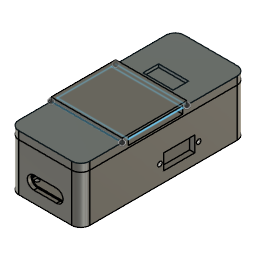
IMU (Autodesk Fusion 360 design; units mm, degrees)
Autodesk Fusion 360 part; units mm, degrees
sketch "草图1" plane through (0, 0, 0) normal (0, 0, 1) x (1, 0, 0)
  line L0 (-10, 20) -> (10, 20)
  line L1 (10, 20) -> (10, -20)
  line L2 (10, -20) -> (-10, -20)
  line L3 (-10, -20) -> (-10, 20)
  line L4 (0, 20) -> (0, -20) construction
  line L5 (-10, 10) -> (10, 10) construction
  circle A0 centre (-10, 10) radius 1.75
  circle A1 centre (10, 10) radius 1.75
  circle A2 centre (-10, 10) radius 1.25
  circle A3 centre (10, 10) radius 1.25
  line L6 (-10.1, -10) -> (10.1, -10) construction
  circle A4 centre (-10.1, -10) radius 2.5
  circle A5 centre (10.1, -10) radius 2.5
  circle A6 centre (0, -20) radius 1.25
  circle A7 centre (0, -20) radius 1.75
  circle A8 centre (0, 20) radius 1.75
  line L7 (-6, 18.2) -> (6, 18.2)
  line L8 (6, 18.2) -> (6, 13.2)
  line L9 (6, 13.2) -> (-6, 13.2)
  line L10 (-6, 13.2) -> (-6, 18.2)
  dimension "d1" = 20
  dimension "d2" = 40
  dimension "d4" = 20
  dimension "d5" = 10
  dimension "d6" = 20
  dimension "d7" = 10
  dimension "d8" = 3.5
  dimension "d9" = 3.5
  dimension "d10" = 2.5
  dimension "d11" = 2.5
  dimension "d12" = 20.2
  dimension "d13" = 10.1
  dimension "d14" = 5
  dimension "d15" = 5
  dimension "d16" = 10
  dimension "d17" = 2.5
  dimension "d18" = 3.5
  dimension "d19" = 3.5
  dimension "d20" = 12
  dimension "d21" = 5
  dimension "d22" = 6
  dimension "d23" = 1.8
  constraint horizontal L0
  constraint vertical L1
  constraint horizontal L2
  constraint vertical L3
  constraint midpoint L0 L4.start
  constraint midpoint L2 L4.end
  constraint horizontal L5
  constraint coincident L5.start A0.centre
  constraint coincident L5.end A1.centre
  constraint concentric A0 A2
  constraint concentric A1 A3
  constraint perpendicular L4 L6
  constraint coincident L6.start A4.centre
  constraint coincident L6.end A5.centre
  constraint coincident L4.end A6.centre
  constraint concentric A6 A7
  constraint coincident L4.start A8.centre
  constraint horizontal L7
  constraint vertical L8
  constraint horizontal L9
  constraint vertical L10
  measures "d1" distance of L0.start L0.end
  measures "d2" distance of L0.start L2.end
  measures "d4" vertical distance of origin L2.end
  measures "d5" distance of L0 L5
  measures "d6" distance of L5.start L5.end
  measures "d7" distance of L4 L5.start
  measures "d8" diameter of A0
  measures "d9" diameter of A1
  measures "d10" diameter of A2
  measures "d11" diameter of A3
  measures "d12" distance of L6.start L6.end
  measures "d13" distance of L4 L6.start
  measures "d14" diameter of A4
  measures "d15" diameter of A5
  measures "d16" distance of L2 L6
  measures "d17" diameter of A6
  measures "d18" diameter of A7
  measures "d19" diameter of A8
  measures "d20" distance of L7.start L7.end
  measures "d21" distance of L7.start L9.end
  measures "d22" distance of L4 L10
  measures "d23" distance of L0 L7
extrude "拉伸1" add sketch "草图1" along normal blind 3 contours L0 L1 L2 L3 A0 A1 A4 A5 A7 A8 | L1 A1 A3 | L1 A1 A3 | L3 A0 A2 | L3 A0 A2 | L2 A6 A7 | L2 A6 A7 makes body 1
extrude "拉伸2" add sketch "草图1" along normal blind 10 contours L7 L8 L9 L10 bodies 1
sketch "草图2" plane through (0, 0, 0) normal (0, 0, 1) x (1, 0, 0)
  line L0 (-12, 21) -> (12, 21)
  line L1 (12, 21) -> (12, -23)
  line L2 (12, -23) -> (-12, -23)
  line L3 (-12, -23) -> (-12, 21)
  circle A0 centre (-10, 10) radius 1.0823
  circle A1 centre (10, 10) radius 1.0591
  circle A2 centre (-10.1, -10) radius 2.4042
  circle A3 centre (10.1, -10) radius 2.4166
  circle A4 centre (0, -20) radius 1.1585
  line L4 (-10, 20) -> (10, 20)
  line L5 (10, 20) -> (10, -20)
  line L6 (10, -20) -> (-10, -20)
  line L7 (-10, -20) -> (-10, 20)
  line L8 (10.3, -20.3) -> (-10.3, -20.3)
  line L9 (-10.3, -20.3) -> (-10.3, 20.3)
  line L10 (-10.3, 20.3) -> (10.3, 20.3)
  line L11 (10.3, 20.3) -> (10.3, -20.3)
  line L12 (-13.1165, -25.5623) -> (-13.1165, 25.5623)
  line L13 (13.1165, 25.5623) -> (13.1165, -25.5623)
  line L14 (13.1165, -25.5623) -> (-13.1165, 25.5623) construction
  line L15 (-13.1165, -25.5623) -> (13.1165, 25.5623) construction
  line L16 (-13.1165, 22.0321) -> (13.1165, 22.0321)
  line L17 (-13.1165, -23.5106) -> (13.1165, -23.5106)
  dimension "d28" = -0.3
  constraint horizontal L0
  constraint vertical L1
  constraint horizontal L2
  constraint vertical L3
  constraint horizontal L4
  constraint vertical L5
  constraint horizontal L6
  constraint vertical L7
  constraint parallel L12 L13
  constraint coincident L14 origin
  constraint coincident L15 origin
  constraint coincident L12 L16.start
  constraint coincident L13 L16.end
  constraint perpendicular L13 L16
  constraint coincident L12 L17.start
  constraint coincident L13 L17.end
  constraint perpendicular L13 L17
extrude "拉伸3" add sketch "草图2" against normal blind 1.5 separate body contours L0 L1 L3 A0 A1 A2 A3 L9 L10 L11 | L3 A2 L9 | L1 A3 L11 | L1 L2 L3 A2 A3 A4 L8 L9 L11 | A0 A2 L7 L9 | A2 L7 L9 | A3 L5 L11 | A1 A3 L5 L11 | A2 A4 L6 L7 L8 L9 | A0 A1 A2 A3 A4 L4 L5 L6 L7 | A2 L7 | A0 L7 L9 | A0 L9 | A3 A4 L5 L6 L8 L11 | A3 L5 | A1 L11 | A1 L5 L11 | A0 L7 | A0 A1 L4 L5 L7 L9 L10 L11 | A1 L5 | A4 L8 | A4 L6 L8 | A4 L6 makes body 2
extrude "拉伸4" add sketch "草图2" along normal blind 1 contours L3 A2 L9 | L1 A3 L11 | A2 L7 L9 | A3 L5 L11 | A2 L7 | A0 L7 L9 | A0 L9 | A3 L5 | A1 L11 | A1 L5 L11 | A0 L7 | A1 L5 | A4 L8 | A4 L6 L8 | A4 L6 bodies 2
extrude "拉伸5" add sketch "草图2" along normal blind 6 and the other way blind 1.5 contours L3 A2 | L1 A3 | L12 L13 L16 L17 bodies 2
extrude "拉伸6" add 5 faces at (-10.521, -9.8562, 1) (0.8928, -19.8469, 1) (9.1946, -9.4156, 1) (10.2131, 9.9372, 1) (-10.1804, 10.3124, 1) along direction (0, 0, 1) blind 0.5 on bodies 2 bodies 2
sketch "草图3" plane through (0, 21, 0) normal (0, -1, 0) x (1, 0, 0)
  line L0 (-12, 0) -> (12, 0)
  line L1 (12, 0) -> (12, 6)
  line L2 (12, 6) -> (-12, 6)
  line L3 (-12, 6) -> (-12, 0)
  line L4 (0, 6) -> (0, 0) construction
  line L5 (-12, 6) -> (-11, 4.5)
  line L6 (-11, 4.5) -> (-12, 4.5)
  line L7 (11, 4.5) -> (12, 4.5)
  line L8 (12, 6) -> (11, 4.5)
  constraint midpoint L2 L4.start
  constraint coincident L4.end origin
  constraint coincident L2.end L3.start
  constraint coincident L3 L6.end
  constraint perpendicular L3 L6
  constraint symmetric L4 L2.end L1.end
  constraint symmetric L4 L5.end L7.start
  constraint symmetric L4 L6.end L7.end
extrude "拉伸7" add sketch "草图3" along normal blind 41 contours L3 L5 L6 | L1 L7 L8 bodies 2
extrude "拉伸8" cut sketch "草图3" along normal blind 12 contours L3 L5 L6 | L1 L7 L8 bodies 2
extrude "拉伸9" cut 2 faces at (-11.6667, -20, 5) (11.6667, -20, 5) along direction (0, 1, 0) blind 9 on bodies 2 bodies 2
sketch "草图4" plane through (0, 0, 6) normal (0, 0, 1) x (-1, 0, 0)
  line L0 (-12, 23) -> (12, 23)
  line L1 (12, 23) -> (12, 11)
  line L2 (12, 11) -> (12, -9)
  line L3 (12, -9) -> (12, -21)
  line L4 (12, -21) -> (-12, -21)
  line L5 (-12, -21) -> (-12, -9)
  line L6 (-12, -9) -> (-12, 11)
  line L7 (-12, 11) -> (-12, 23)
  line L8 (13.1165, -22.0321) -> (13.1165, 23.5106)
  line L9 (13.1165, 23.5106) -> (-13.1165, 23.5106)
  line L10 (-13.1165, 23.5106) -> (-13.1165, -22.0321)
  line L11 (-13.1165, -22.0321) -> (13.1165, -22.0321)
  line L12 (13.1165, -10.0589) -> (12, -10.0589)
  line L13 (12, -10.0589) -> (12, -9)
  line L14 (12, -9) -> (13.1165, -9)
  line L15 (13.1165, -9) -> (13.1165, -10.0589)
  line L16 (-12, -10) -> (-13.1165, -10)
  line L17 (-13.1165, -10) -> (-13.1165, -8.9928)
  line L18 (-13.1165, -8.9928) -> (-12, -8.9928)
  line L19 (-12, -8.9928) -> (-12, -10)
  line L20 (13.1165, 10.9187) -> (12, 10.9187)
  line L21 (12, 10.9187) -> (12, 12)
  line L22 (12, 12) -> (13.1165, 12)
  line L23 (13.1165, 12) -> (13.1165, 10.9187)
  line L24 (-12, 11) -> (-13.1165, 11)
  line L25 (-13.1165, 11) -> (-13.1165, 12.0535)
  line L26 (-13.1165, 12.0535) -> (-12, 12.0535)
  line L27 (-12, 12.0535) -> (-12, 11)
  constraint horizontal L12
  constraint vertical L13
  constraint horizontal L14
  constraint vertical L15
  constraint coincident L2.end L3.start
  constraint coincident L8 L12.start
  constraint horizontal L16
  constraint vertical L17
  constraint horizontal L18
  constraint vertical L19
  constraint coincident L10 L17.end
  constraint coincident L5 L16.start
  constraint horizontal L20
  constraint vertical L21
  constraint horizontal L22
  constraint vertical L23
  constraint coincident L1 L21.end
  constraint coincident L8 L20.start
  constraint horizontal L24
  constraint vertical L25
  constraint horizontal L26
  constraint vertical L27
  constraint coincident L10 L25.end
  constraint coincident L6.end L7.start
extrude "拉伸10" cut sketch "草图4" against normal blind 3 contours L7 L10 L24 L25 L26 L27 | L1 L2 L8 L20 L21 L22 L23 | L5 L6 L10 L16 L17 L18 L19 | L3 L8 L12 L13 L14 L15 bodies 2
sketch "草图5" plane through (0, 0, 0) normal (0, 0, 1) x (1, 0, 0)
  line L0 (12, 21) -> (-12, 21)
  line L1 (-12, 21) -> (-12, -23)
  line L2 (12, -23) -> (12, 21)
  line L3 (11.6151, 20.6151) -> (-11.6151, 20.6151)
  line L4 (-11.6151, 20.6151) -> (-11.6151, -22.6151)
  line L5 (-11.6151, -22.6151) -> (11.6151, -22.6151)
  line L6 (11.6151, -22.6151) -> (11.6151, 20.6151)
  line L7 (6, 18.2) -> (-6, 18.2)
  line L8 (-6, 18.2) -> (-6, 13.2)
  line L9 (-6, 13.2) -> (6, 13.2)
  line L10 (6, 13.2) -> (6, 18.2)
  line L11 (-6.4291, 18.6291) -> (-6.4291, 12.7709)
  line L12 (-6.4291, 12.7709) -> (6.4291, 12.7709)
  line L13 (6.4291, 12.7709) -> (6.4291, 18.6291)
  line L14 (6.4291, 18.6291) -> (-6.4291, 18.6291)
  point P0 (12, 21)
  point P1 (-12, -23)
  point P2 (6, 18.2)
  point P3 (-6, 13.2)
  dimension "d47" = -0.3849
  dimension "d48" = 0.4291
  constraint horizontal L0
  constraint vertical L1
  constraint vertical L2
  constraint coincident P1 L1.end
  constraint coincident P0 L0.start
  constraint horizontal L7
  constraint vertical L8
  constraint horizontal L9
  constraint vertical L10
  constraint coincident P3 L8.end
  constraint coincident P2 L7.start
extrude "拉伸11" add sketch "草图5" along normal blind 2 separate body contours L3 L4 L5 L6 makes body 3
move_body "移动1" bodies 3 to x (1, 0, 0) y (0, 1, 0) z (0, 0, 1) at (0, 0, 2)
move_body "移动2" bodies 3 to x (1, 0, 0) y (0, 1, 0) z (0, 0, 1) at (0, 0, 13)
extrude "拉伸12" cut 1 faces at (2.143, -10.8198, 17) along direction (0, 0, -1) blind 0.7 on bodies 3 bodies 3
move_body "移动3" bodies 3 to x (1, 0, 0) y (0, 1, 0) z (0, 0, 1) at (0, 0, -12)
extrude "拉伸13" add 1 faces at (11.6151, -8.205, 3.4333) along direction (1, 0, 0) blind 0.3 on bodies 3 bodies 3
extrude "拉伸14" cut 4 faces at (-12.3722, 9.353, 3) (-12.3722, -11.6396, 3) (12.3722, -11.7023, 3) (12.7443, 9.3286, 3) along direction (0, 0, -1) blind 3 on bodies 2 bodies 2
sketch "草图6" plane through (0, 0, 4.3) normal (0, 0, 1) x (-1, 0, 0)
  line L0 (6.4291, -18.6291) -> (-6.4291, -18.6291)
  line L1 (-6.4291, -18.6291) -> (-6.4291, -12.7709)
  line L2 (-6.4291, -12.7709) -> (6.4291, -12.7709)
  line L3 (6.4291, -12.7709) -> (6.4291, -18.6291)
  line L4 (-11.9151, -20.6151) -> (11.6151, -20.6151)
  line L5 (11.6151, -20.6151) -> (11.6151, 22.6151)
  line L6 (11.6151, 22.6151) -> (-11.9151, 22.6151)
  line L7 (-11.9151, 22.6151) -> (-11.9151, -20.6151)
  line L8 (9, -8) -> (-8.9143, -8)
  line L9 (-8.9143, -8) -> (-8.9143, 14.5)
  line L10 (-8.9143, 14.5) -> (9, 14.5)
  line L11 (9, 14.5) -> (9, -8)
  dimension "d57" = 22.5
  constraint horizontal L8
  constraint vertical L9
  constraint horizontal L10
  constraint vertical L11
  measures "d57" distance of L8.start L10.end
extrude "拉伸15" add sketch "草图6" along normal blind 6.5 contours L8 L9 L10 L11 bodies 3
fillet "圆角1" radius 1 8 edges at (-0.0428, 8, 10.8) (-0.0428, -14.5, 10.8) (-9, -3.25, 10.8) (8.9143, -3.25, 10.8) (-9, 8, 7.55) (-9, -14.5, 7.55) (8.9143, -14.5, 7.55) (8.9143, 8, 7.55) on bodies 3
sketch "草图7" plane through (-9, 0, 0) normal (-1, 0, 0) x (0, -1, 0)
  line L0 (13.5, 4.3) -> (13.5, 9.8)
  line L1 (13.5, 9.8) -> (-7, 9.8)
  line L2 (-7, 9.8) -> (-7, 4.3)
  line L3 (-7, 4.3) -> (13.5, 4.3)
  line L4 (-7, 9.8) -> (13.5, 9.8)
  line L5 (13.5, 9.8) -> (13.5, 6.8)
  line L6 (13.5, 6.8) -> (-7, 6.8)
  line L7 (-7, 6.8) -> (-7, 9.8)
  dimension "d62" = 3
  constraint horizontal L4
  constraint vertical L5
  constraint horizontal L6
  constraint vertical L7
  constraint coincident L0 L5.end
  constraint coincident L1.end L2.start
  measures "d62" distance of L1.end L6.end
extrude "拉伸16" cut sketch "草图7" against normal blind 20 contours L0 L1 L2 L4 L5 L6 L7 bodies 3
fillet "圆角2" radius 0.5 4 edges at (-9, -3.25, 9.8) (-9, -3.25, 6.8) (8.9143, -3.25, 9.8) (8.9143, -3.25, 6.8) on bodies 3
sketch "草图8" plane through (0, 0, 0) normal (0, 0, 1) x (1, 0, 0)
  line L0 (75, 20) -> (98.5, 20)
  line L1 (98.5, 20) -> (98.5, -41)
  line L2 (98.5, -41) -> (75, -41)
  line L3 (75, -41) -> (75, 20)
  line L4 (75, 19) -> (98.5, 19)
  line L5 (74, 20) -> (74, -42)
  line L6 (74, -42) -> (99.5, -42)
  line L7 (99.5, -42) -> (99.5, 20)
  line L8 (99.5, 20) -> (74, 20)
  dimension "d67" = 23.5
  dimension "d68" = 61
  constraint horizontal L0
  constraint vertical L1
  constraint horizontal L2
  constraint vertical L3
  constraint coincident L3 L4.start
  constraint coincident L1 L4.end
  constraint perpendicular L1 L4
  constraint perpendicular L0 L5
  constraint perpendicular L5 L6
  constraint perpendicular L6 L7
  constraint perpendicular L5 L8
  measures "d67" distance of L0.start L0.end
  measures "d68" distance of L0.start L2.end
extrude "拉伸17" add sketch "草图8" along normal blind 21 separate body contours L0 L1 L3 L4 L8 | L1 L2 L3 L5 L6 L7 L8 makes body 4
extrude "拉伸18" add sketch "草图8" along normal blind 2 contours L1 L2 L3 L4 bodies 4
sketch "草图9" plane through (0, 0, 0) normal (0, 1, 0) x (1, 0, 0)
  line L0 (105, -1) -> (122.5, -1)
  line L1 (122.5, -1) -> (122.5, 0)
  line L2 (122.5, 0) -> (105, 0)
  line L3 (105, 0) -> (105, -1)
  line L4 (109.35, -3.9902) -> (118.15, -3.9902)
  arc A0 (118.15, -3.9902) -> (118.15, -0.9902) centre (118.15, -2.4902) ccw
  line L5 (118.15, -0.9902) -> (109.35, -0.9902)
  arc A1 (109.35, -0.9902) -> (109.35, -3.9902) centre (109.35, -2.4902) ccw
  line L6 (109.35, -2.4902) -> (118.15, -2.4902) construction
  point P0 (113.75, -1)
  point P1 (113.75, -2.4902)
  dimension "d73" = 17.5
  dimension "d76" = 3
  constraint horizontal L0
  constraint vertical L1
  constraint horizontal L2
  constraint vertical L3
  constraint midpoint L0 P0
  constraint tangent L4 A0
  constraint tangent A0 L5
  constraint parallel L4 L5
  constraint tangent L5 A1
  constraint tangent L4 A1
  constraint parallel L0 L6
  constraint midpoint L6 P1
  measures "d73" distance of L0.start L0.end
  measures "d76" diameter of A0
extrude "拉伸19" add sketch "草图9" along normal blind 28 separate body contours L0 L1 L2 L3 A0 L5 A1 | L0 A0 L5 A1 makes body 5
extrude "拉伸20" add sketch "草图9" along normal blind 6.1 and the other way blind 0.7 contours L0 L4 A0 A1 bodies 5
sketch "草图10" plane through (0, 0, 1) normal (0, 0, 1) x (-1, 0, 0)
  line L0 (-118.3209, -6.1) -> (-118.3209, 0)
  line L1 (-118.3209, 0) -> (-122.5, 0)
  line L2 (-122.5, 0) -> (-122.5, -28)
  line L3 (-122.5, -28) -> (-105, -28)
  line L4 (-105, -28) -> (-105, 0)
  line L5 (-105, 0) -> (-109.1791, 0)
  line L6 (-109.1791, 0) -> (-109.1791, -6.1)
  line L7 (-109.1791, -6.1) -> (-118.3209, -6.1)
  line L8 (-120.75, -1.9) -> (-106.75, -1.9)
  circle A0 centre (-106.75, -1.9) radius 0.8
  circle A1 centre (-120.75, -1.9) radius 0.8
  line L9 (-105, 0) -> (-122.5, 0)
  dimension "d81" = 14
  dimension "d82" = 1.75
  dimension "d83" = 1.6
  dimension "d84" = 1.6
  dimension "d87" = 17.5
  dimension "d91" = 1.9
  constraint perpendicular L4 L8
  constraint coincident L8.end A0.centre
  constraint coincident L8.start A1.centre
  measures "d81" distance of L8.start L8.end
  measures "d82" distance of L2 L8.start
  measures "d83" diameter of A0
  measures "d84" diameter of A1
  measures "d87" distance of L2.end L3.end
  measures "d91" distance of L8 L9
extrude "拉伸21" cut sketch "草图10" against normal blind 1.6 contours A0 | A1 bodies 5
sketch "草图11" plane through (0, 0, 2) normal (0, 0, 1) x (-1, 0, 0)
  line L0 (-75, -19) -> (-75, 41)
  line L1 (-75, 41) -> (-98.5, 41)
  line L2 (-98.5, 41) -> (-98.5, -19)
  line L3 (-98.5, -19) -> (-75, -19)
  line L4 (-86.75, 41) -> (-86.75, -19) construction
  line L5 (-95.5, 41) -> (-78, 41)
  line L6 (-78, 41) -> (-78, 22.3)
  line L7 (-78, 22.3) -> (-95.5, 22.3)
  line L8 (-95.5, 22.3) -> (-95.5, 41)
  line L9 (-93.75, 39.1) -> (-79.75, 39.1) construction
  circle A0 centre (-93.75, 39.1) radius 0.5239
  circle A1 centre (-79.75, 39.1) radius 0.5069
  dimension "d88" = 17.5
  dimension "d89" = 18.7
  dimension "d90" = 8.75
  dimension "d92" = 14
  dimension "d93" = 1.75
  dimension "d94" = 1.9
  constraint midpoint L1 L4.start
  constraint midpoint L3 L4.end
  constraint horizontal L5
  constraint vertical L6
  constraint horizontal L7
  constraint vertical L8
  constraint coincident L1 L5.start
  constraint parallel L1 L9
  constraint coincident L9.start A0.centre
  constraint coincident L9.end A1.centre
  measures "d88" distance of L5.start L5.end
  measures "d89" distance of L5.start L7.end
  measures "d90" distance of L4 L8
  measures "d92" distance of L9.start L9.end
  measures "d93" distance of L8 L9.start
  measures "d94" distance of L5 L9
extrude "拉伸22" add sketch "草图11" along normal blind 2.5 contours L1 L5 L6 L7 L8 bodies 4
thread "螺纹1" "ISO Metric profile 2.0 M2x0.4 M2x0.4 6H" major diameter 2.074 minor diameter 1.623 pitch 0.4 angle 60 resizes the face on face at (93.4658, -39.5401, 3.6667) on face at (79.4146, -39.48, 3.6667) on bodies 4
move_body "移动4" bodies 5 to x (1, 0, 0) y (0, 1, 0) z (0, 0, 1) at (-26.9998, -40.9666, 1.427)
move_body "移动5" bodies 5 to x (1, 0, 0) y (0, 1, 0) z (0, 0, 1) at (0, 0, 3.1)
sketch "草图12" plane through (0, -41, 0) normal (0, 1, 0) x (-1, 0, 0)
  line L0 (-78, 4.5) -> (-78, 2)
  line L1 (-78, 2) -> (-75, 2)
  line L2 (-75, 2) -> (-75, 21)
  line L3 (-75, 21) -> (-98.5, 21)
  line L4 (-98.5, 21) -> (-98.5, 2)
  line L5 (-98.5, 2) -> (-95.5, 2)
  line L6 (-95.5, 2) -> (-95.5, 4.5)
  line L7 (-95.5, 4.5) -> (-78, 4.5)
  arc A0 through (-91.1502, 8.5172, -0.6666) (-92.6478, 7.1028, -0.6666) (-91.3212, 5.527, -0.6666)
  arc A1 through (-82.1793, 5.527, -0.6666) (-80.8527, 7.1028, -0.6666) (-82.3503, 8.5172, -0.6666)
  line L8 (-91.1502, 8.5172, -0.6666) -> (-82.3503, 8.5172, -0.6666)
  line L9 (-91.3212, 5.527, -0.6666) -> (-82.1793, 5.527, -0.6666)
  line L10 (-91.1503, 5.3759) -> (-82.35, 5.3759)
  arc A2 (-82.35, 5.3759) -> (-82.35, 8.6585) centre (-82.35, 7.0172) ccw
  line L11 (-82.35, 8.6585) -> (-91.1503, 8.6585)
  arc A3 (-91.1503, 8.6585) -> (-91.1503, 5.3759) centre (-91.1503, 7.0172) ccw
  line L12 (-91.1503, 7.0172) -> (-82.35, 7.0172) construction
  line L13 (-82.35, 9.5343) -> (-91.1503, 9.5343)
  arc A4 (-91.1503, 9.5343) -> (-91.1503, 4.5) centre (-91.1503, 7.0172) ccw
  line L14 (-91.1503, 4.5) -> (-82.35, 4.5)
  arc A5 (-82.35, 4.5) -> (-82.35, 9.5343) centre (-82.35, 7.0172) ccw
  line L15 (-82.35, 7.0172) -> (-91.1503, 7.0172) construction
  constraint tangent L10 A2
  constraint tangent A2 L11
  constraint parallel L10 L11
  constraint tangent L11 A3
  constraint tangent L10 A3
  constraint horizontal L12
  constraint tangent L13 A4
  constraint tangent A4 L14
  constraint parallel L13 L14
  constraint tangent L14 A5
  constraint tangent L13 A5
  constraint coincident A3.centre L12.start
  constraint parallel L12 L15
  constraint coincident A2.centre L12.end
extrude "拉伸23" cut sketch "草图12" against normal blind 3 contours L10 A2 L11 A3 bodies 4
sketch "草图13" plane through (0, -42, 0) normal (0, -1, 0) x (1, 0, 0)
  line L0 (91.1503, 5.3759) -> (82.35, 5.3759)
  arc A0 (82.35, 8.6585) -> (82.35, 5.3759) centre (82.35, 7.0172) ccw
  line L1 (82.35, 8.6585) -> (91.1503, 8.6585)
  arc A1 (91.1503, 5.3759) -> (91.1503, 8.6585) centre (91.1503, 7.0172) ccw
  line L2 (74, 0) -> (99.5, 0)
  line L3 (99.5, 0) -> (99.5, 21)
  line L4 (99.5, 21) -> (74, 21)
  line L5 (74, 21) -> (74, 0)
  line L6 (82.35, 4.5) -> (91.1503, 4.5)
  arc A2 (91.1503, 4.5) -> (91.1503, 9.5343) centre (91.1503, 7.0172) ccw
  line L7 (91.1503, 9.5343) -> (82.35, 9.5343)
  arc A3 (82.35, 9.5343) -> (82.35, 4.5) centre (82.35, 7.0172) ccw
  line L8 (82.35, 7.0172) -> (91.1503, 7.0172) construction
  constraint tangent L6 A2
  constraint tangent A2 L7
  constraint parallel L6 L7
  constraint tangent L7 A3
  constraint tangent L6 A3
  constraint coincident A1.centre A2.centre
  constraint horizontal L8
  constraint coincident A0.centre A3.centre
extrude "拉伸24" cut sketch "草图13" against normal blind 0.5 contours L6 A2 L7 A3 bodies 4
sketch "草图14" plane through (0, 0, 0) normal (0, 0, 1) x (1, 0, 0)
  line L0 (50, 5) -> (70, 5)
  line L1 (70, 5) -> (70, -47.6)
  line L2 (70, -47.6) -> (50, -47.6)
  line L3 (50, -47.6) -> (50, 5)
  circle A0 centre (52, 3) radius 1.05
  circle A1 centre (68, 3) radius 1.05
  line L4 (55, 5) -> (65, 5)
  line L5 (65, 5) -> (65, 12.7)
  line L6 (65, 12.7) -> (55, 12.7)
  line L7 (55, 12.7) -> (55, 5)
  dimension "d103" = 20
  dimension "d104" = 52.6
  dimension "d105" = 2.1
  dimension "d106" = 2.1
  dimension "d107" = 2
  dimension "d108" = 2
  dimension "d109" = 2
  dimension "d110" = 2
  dimension "d111" = 10
  dimension "d112" = 7.7
  dimension "d113" = 5
  constraint horizontal L0
  constraint vertical L1
  constraint horizontal L2
  constraint vertical L3
  constraint horizontal L4
  constraint vertical L5
  constraint horizontal L6
  constraint vertical L7
  constraint coincident L0 L4.start
  measures "d103" distance of L0.start L0.end
  measures "d104" distance of L0.start L2.end
  measures "d105" diameter of A0
  measures "d106" diameter of A1
  measures "d107" distance of L0 A1.centre
  measures "d108" distance of L0 A0.centre
  measures "d109" distance of L3 A0.centre
  measures "d110" distance of L1 A1.centre
  measures "d111" distance of L4.start L4.end
  measures "d112" distance of L4.start L6.end
  measures "d113" distance of L3 L7
extrude "拉伸25" add sketch "草图14" along normal blind 1.4 separate body contours L0 L1 L2 L3 L4 makes body 6
extrude "拉伸26" add sketch "草图14" along normal blind 4.2 and the other way blind 0.6 contours L0 L4 L5 L6 L7 bodies 6
sketch "草图15" plane through (0, 0, 1.4) normal (0, 0, 1) x (-1, 0, 0)
  circle A0 centre (-68, -3) radius 1.05
  circle A1 centre (-52, -3) radius 1.05
  line L0 (-70, -5) -> (-65, -5)
  line L1 (-65, -5) -> (-55, -5)
  line L2 (-55, -5) -> (-50, -5)
  line L3 (-50, -5) -> (-50, 47.6)
  line L4 (-50, 47.6) -> (-70, 47.6)
  line L5 (-70, 47.6) -> (-70, -5)
  line L6 (-54.7, 2.1) -> (-65.3, 2.1)
  line L7 (-65.3, 2.1) -> (-65.3, 7.1)
  line L8 (-65.3, 7.1) -> (-54.7, 7.1)
  line L9 (-54.7, 7.1) -> (-54.7, 2.1)
  line L10 (-50, -5) -> (-70, -5)
  line L11 (-70, -5) -> (-70, 47.6)
  line L12 (-50, 47.6) -> (-50, -5)
  dimension "d120" = 10.6
  dimension "d121" = 5
  dimension "d122" = 7.1
  dimension "d123" = 4.7
  dimension "d124" = 4.7
  constraint horizontal L6
  constraint vertical L7
  constraint horizontal L8
  constraint vertical L9
  measures "d120" distance of L6.start L6.end
  measures "d121" distance of L6.start L8.end
  measures "d122" distance of L6 L10
  measures "d123" distance of L7 L11
  measures "d124" distance of L9 L12
extrude "拉伸27" add sketch "草图15" along normal blind 8.4 contours L6 L7 L8 L9 bodies 6
move_body "移动6" bodies 6 to x (1, 0, 0) y (0, 1, 0) z (0, 0, 1) at (27, 8, 11)
sketch "草图16" plane through (0, -41, 0) normal (0, 1, 0) x (-1, 0, 0)
  line L0 (-98.5, 21) -> (-98.5, 2) construction
  line L1 (-75, 2) -> (-75, 21) construction
  line L2 (-98.5, 11) -> (-75, 11) construction
  line L3 (-98.5, 2) -> (-95.5, 2) construction
  line L4 (-98.5, 11) -> (-96.1003, 11)
  line L5 (-96.1003, 11) -> (-96.1003, 9)
  line L6 (-96.1003, 9) -> (-98.5, 9)
  line L7 (-98.5, 9) -> (-98.5, 11)
  line L8 (-98.5, 12.5) -> (-96.1003, 12.5)
  line L9 (-96.1003, 12.5) -> (-96.1003, 14.5)
  line L10 (-96.1003, 14.5) -> (-98.5, 14.5)
  line L11 (-98.5, 14.5) -> (-98.5, 12.5)
  line L12 (-75, 11) -> (-77.5, 11)
  line L13 (-77.5, 11) -> (-77.5, 9)
  line L14 (-77.5, 9) -> (-75, 9)
  line L15 (-75, 9) -> (-75, 11)
  line L16 (-75, 12.5) -> (-77.5, 12.5)
  line L17 (-77.5, 12.5) -> (-77.5, 14.5)
  line L18 (-77.5, 14.5) -> (-75, 14.5)
  line L19 (-75, 14.5) -> (-75, 12.5)
  dimension "d127" = 9
  dimension "d128" = 2
  dimension "d129" = 2
  dimension "d130" = 1.5
  dimension "d138" = 1.5
  constraint coincident L0 L2.start
  constraint coincident L1 L2.end
  constraint perpendicular L1 L2
  constraint horizontal L4
  constraint vertical L5
  constraint horizontal L6
  constraint vertical L7
  constraint horizontal L8
  constraint vertical L9
  constraint horizontal L10
  constraint vertical L11
  constraint coincident L0 L8.start
  constraint horizontal L12
  constraint vertical L13
  constraint horizontal L14
  constraint vertical L15
  constraint horizontal L16
  constraint vertical L17
  constraint horizontal L18
  constraint vertical L19
  constraint coincident L1 L16.start
  measures "d127" distance of L2 L3
  measures "d128" distance of L2.start L6.end
  measures "d129" distance of L8.start L10.end
  measures "d130" distance of L2 L8
  measures "d138" distance of L12 L16
extrude "拉伸28" add sketch "草图16" along normal blind 3 bodies 4
move_face "偏移面1" offset -1 4 faces at (85.2834, -41.1667, 8.6585) (91.7878, -41.1667, 5.5047) (81.7886, -41.3333, 5.4748) (88.2168, -41.1667, 5.3759) on bodies 4
extrude "拉伸29" add 4 faces at (97.7001, -38, 13.8333) (96.9002, -38, 9.6667) (75.8333, -38, 13.1667) (76.6667, -38, 10.3333) along direction (0, 1, 0) blind 1 on bodies 4 bodies 4
extrude "拉伸30" cut 2 faces at (97.7001, -37, 13.8333) (75.8333, -37, 13.1667) along direction (0, -1, 0) blind 4 on bodies 4 bodies 4
extrude "拉伸31" add sketch "草图16" along normal blind 4 contours L8 L9 L10 L11 | L16 L17 L18 L19 bodies 4
sketch "草图17" plane through (0, 0, 2) normal (0, 0, 1) x (-1, 0, 0)
  line L0 (-78, 41) -> (-78, 22.3)
  line L1 (-78, 22.3) -> (-95.5, 22.3)
  line L2 (-95.5, 22.3) -> (-95.5, 41)
  line L3 (-95.5, 41) -> (-98.5, 41)
  line L4 (-98.5, 41) -> (-98.5, -19)
  line L5 (-98.5, -19) -> (-75, -19)
  line L6 (-75, -19) -> (-75, 41)
  line L7 (-75, 41) -> (-78, 41)
  circle A0 centre (-95, -11) radius 1.05
  circle A1 centre (-79, -11) radius 1.05
  line L8 (-98.5, -8.2706, -2) -> (-94.3, -8.2706, -2)
  line L9 (-93.2, -9.3706, -2) -> (-93.2, -11.4, -2)
  line L10 (-94.3, -12.5, -2) -> (-98.5, -12.5, -2)
  line L11 (-98.5, -12.5, -2) -> (-98.5, -8.2706, -2)
  line L12 (-98.5, -20, -2) -> (-98.5, 41, -2)
  line L13 (-75, -8.2706, -2) -> (-80.3, -8.2706, -2)
  line L14 (-81.4, -9.3706, -2) -> (-81.4, -11.4, -2)
  line L15 (-80.3, -12.5, -2) -> (-75, -12.5, -2)
  line L16 (-75, -12.5, -2) -> (-75, -8.2706, -2)
  line L17 (-75, 41, -2) -> (-75, -20, -2)
  arc A2 through (-93.2, -9.3706, -2) (-93.5222, -8.5928, -2) (-94.3, -8.2706, -2)
  arc A3 through (-94.3, -12.5, -2) (-93.5222, -12.1778, -2) (-93.2, -11.4, -2)
  arc A4 through (-80.3, -8.2706, -2) (-81.0778, -8.5928, -2) (-81.4, -9.3706, -2)
  arc A5 through (-81.4, -11.4, -2) (-81.0778, -12.1778, -2) (-80.3, -12.5, -2)
  dimension "d141" = 1.1
extrude "拉伸32" add sketch "草图17" along normal blind 11 contours L8 L9 L10 L11 L12 A2 A3 | L13 L14 L15 L16 L17 A4 A5 in plane through (0, 0, 0) normal (0, 0, 1) bodies 4
extrude "拉伸33" cut sketch "草图17" along normal blind 9 contours A0 | A1 bodies 4
thread "螺纹2" "ISO Metric profile 2.0 M2x0.25 M2x0.25 6H" major diameter 2.0555 minor diameter 1.7694 pitch 0.25 angle 60 resizes the face on face at (95.837, 11.634, 8) on face at (79.837, 11.634, 8) on bodies 4
sketch "草图18" plane through (0, 19, 0) normal (0, -1, 0) x (1, 0, 0)
  line L0 (75, 2) -> (98.5, 2)
  line L1 (98.5, 2) -> (98.5, 21)
  line L2 (98.5, 21) -> (75, 21)
  line L3 (75, 21) -> (75, 2)
  line L4 (82, 12.4) -> (92, 12.4)
  line L5 (92, 12.4) -> (92, 15.2)
  line L6 (92, 15.2) -> (82, 15.2)
  line L7 (82, 15.2) -> (82, 12.4)
  line L8 (81.8034, 12.2034) -> (92.1966, 12.2034)
  line L9 (92.1966, 12.2034) -> (92.1966, 15.3966)
  line L10 (92.1966, 15.3966) -> (81.8034, 15.3966)
  line L11 (81.8034, 15.3966) -> (81.8034, 12.2034)
  dimension "d148" = 0.1966
extrude "拉伸34" cut sketch "草图18" against normal blind 2.5 contours L4 L5 L6 L7 | L8 L9 L10 L11 bodies 4
move_face "偏移面2" offset -0.4 4 faces at (88.7322, 19.3333, 15.3966) (81.8034, 19.3333, 14.3322) (85.2678, 19.3333, 12.2034) (92.1966, 19.3333, 13.2678) on bodies 4
sketch "草图19" plane through (0, 0, 21) normal (0, 0, 1) x (-1, 0, 0)
  line L0 (-75, 41) -> (-75, -19)
  line L1 (-75, -19) -> (-98.5, -19)
  line L2 (-98.5, -19) -> (-98.5, 41)
  line L3 (-98.5, 41) -> (-75, 41)
  line L4 (-99.5, -20) -> (-74, -20)
  line L5 (-74, -20) -> (-74, 42)
  line L6 (-74, 42) -> (-99.5, 42)
  line L7 (-99.5, 42) -> (-99.5, -20)
  circle A0 centre (-95.5585, 38) radius 2.05
  circle A1 centre (-77.7898, -16.3705) radius 2.05
  line L8 (-75, -19) -> (-81, -19)
  line L9 (-81, -19) -> (-81, -13)
  line L10 (-81, -13) -> (-75, -13)
  line L11 (-75, -13) -> (-75, -19)
  line L12 (-98.5, 41) -> (-92.5, 41)
  line L13 (-92.5, 41) -> (-92.5, 35)
  line L14 (-92.5, 35) -> (-98.5, 35)
  line L15 (-98.5, 35) -> (-98.5, 41)
  point P0 (-96, 38)
  dimension "d152" = 4.1
  dimension "d153" = 4.1
  dimension "d154" = 6
  dimension "d155" = 6
  dimension "d156" = 6
  dimension "d157" = 6
  constraint horizontal L8
  constraint vertical L9
  constraint horizontal L10
  constraint vertical L11
  constraint coincident L0.end L1.start
  constraint horizontal L12
  constraint vertical L13
  constraint horizontal L14
  constraint vertical L15
  constraint coincident L2.end L3.start
  measures "d152" diameter of A0
  measures "d153" diameter of A1
  measures "d154" distance of L0.end L8.end
  measures "d155" distance of L0.end L10.end
  measures "d156" distance of L2.end L12.end
  measures "d157" distance of L2.end L14.end
extrude "拉伸35" add sketch "草图19" against normal blind 3 contours L2 L3 L12 L13 L14 L15 | A0 bodies 4
extrude "拉伸36" add sketch "草图19" against normal blind 3 contours L0 L1 L8 L9 L10 L11 | A1 bodies 4
extrude "拉伸37" cut sketch "草图19" against normal blind 2.1 contours A0 | A1 bodies 4
fillet "圆角3" radius 2.5 2 edges at (92.5, -35, 19.5) (81, 13, 19.5) on bodies 4
extrude "拉伸38" add 1 faces at (99.5, -21.3333, 14) along direction (1, 0, 0) blind 1 on bodies 4 bodies 4
extrude "拉伸39" add 1 faces at (89.0322, 20, 3.9345) along direction (0, 1, 0) blind 1 on bodies 4 bodies 4
extrude "拉伸40" add 1 faces at (74, -21, 14) along direction (-1, 0, 0) blind 1 on bodies 4 bodies 4
extrude "拉伸41" add 1 faces at (85.2833, -42, 17.1781) along direction (0, -1, 0) blind 1 on bodies 4 bodies 4
extrude "拉伸42" cut 1 faces at (99.8333, -19, 21) along direction (0, 0, -1) blind 2.5 on bodies 4 bodies 4
extrude "拉伸43" cut sketch "草图19" against normal blind 3 contours L2 L3 L12 L13 L14 L15 | A0 bodies 4
extrude "拉伸44" cut sketch "草图19" against normal blind 3 contours L0 L1 L8 L9 L10 L11 | A1 bodies 4
extrude "拉伸45" add sketch "草图19" against normal blind 5.5 contours L0 L1 L8 L9 L10 L11 | L2 L3 L12 L13 L14 L15 | A0 | A1 bodies 4
extrude "拉伸46" cut sketch "草图19" against normal blind 2.5 contours L0 L1 L8 L9 L10 L11 | L2 L3 L12 L13 L14 L15 | A0 | A1 bodies 4
extrude "拉伸47" cut sketch "草图19" against normal blind 4.1 contours A0 | A1 bodies 4
extrude "拉伸48" cut 1 faces at (77.4482, 15.575, 16.9) along direction (0, 0, -1) blind 1 on bodies 4 bodies 4
extrude "拉伸49" add 1 faces at (77.4482, 15.575, 15.9) along direction (0, 0, 1) blind 0.4 on bodies 4 bodies 4
extrude "拉伸50" add 1 faces at (77.4482, 15.575, 16.3) along direction (0, 0, 1) blind 0.1 on bodies 4 bodies 4
extrude "拉伸51" cut 1 faces at (95.8082, -38.6361, 16.9) along direction (0, 0, -1) blind 0.5 on bodies 4 bodies 4
fillet "圆角4" radius 2.5 2 edges at (92.5, -35, 17) (81, 13, 17) on bodies 4
sketch "草图20" plane through (0, 0, 18.5) normal (0, 0, 1) x (-1, 0, 0)
  arc A0 (-78.5, -13) -> (-81, -15.5) centre (-78.5, -15.5) ccw
  line L0 (-81, -15.5) -> (-81, -19)
  line L1 (-81, -19) -> (-98.5, -19)
  line L2 (-98.5, -19) -> (-98.5, 35)
  line L3 (-98.5, 35) -> (-95, 35)
  arc A1 (-95, 35) -> (-92.5, 37.5) centre (-95, 37.5) ccw
  line L4 (-92.5, 37.5) -> (-92.5, 41)
  line L5 (-92.5, 41) -> (-75, 41)
  line L6 (-75, 41) -> (-75, -13)
  line L7 (-75, -13) -> (-78.5, -13)
  circle A2 centre (-77.7898, -16.3705) radius 2.05
  circle A3 centre (-95.5585, 38) radius 2.05
  line L8 (-100.5, 43) -> (-100.5, -21)
  line L9 (-100.5, -21) -> (-73, -21)
  line L10 (-73, -21) -> (-73, 43)
  line L11 (-73, 43) -> (-100.5, 43)
extrude "拉伸52" add sketch "草图20" along normal blind 3 separate body makes body 7
extrude "拉伸53" add sketch "草图20" along normal blind 3 contours A0 L0 L1 L2 L3 A1 L4 L5 L6 L7 bodies 7
extrude "拉伸54" add sketch "草图20" along normal blind 3 contours A2 | A3 bodies 7
extrude "拉伸55" cut sketch "草图20" along normal blind 2.1 contours A2 | A3 bodies 7
combine "合并1" operation cut target body 7 tool bodies 6 keep tools
extrude "拉伸56" cut 1 faces at (88.7667, 4.2333, 20.8) along direction (0, 0, 1) blind 14 on bodies 7 bodies 7
move_face "偏移面3" offset -0.5 4 faces at (88.7667, 0.9, 19.5) (92.3, 4.2333, 19.5) (85.2333, 5.9, 19.5) (81.7, 2.5667, 19.5) on bodies 7
extrude "拉伸57" cut 1 faces at (85.1345, 20.3333, 11.8034) along direction (0, 0, -1) blind 2 on bodies 4 bodies 4
sketch "草图21" plane through (98.5, 0, 0) normal (-1, 0, 0) x (0, -1, 0)
  line L0 (35, 15.5) -> (35, 18.5)
  line L1 (35, 18.5) -> (-19, 18.5)
  line L2 (-19, 18.5) -> (-19, 2)
  line L3 (-19, 2) -> (-12.5, 2)
  line L4 (-12.5, 2) -> (-12.5, 11)
  line L5 (-12.5, 11) -> (-8.2706, 11)
  line L6 (-8.2706, 11) -> (-8.2706, 2)
  line L7 (-8.2706, 2) -> (41, 2)
  line L8 (41, 2) -> (41, 9)
  line L9 (41, 9) -> (37, 9)
  line L10 (37, 9) -> (37, 11)
  line L11 (37, 11) -> (41, 11)
  line L12 (41, 11) -> (41, 12.5)
  line L13 (41, 12.5) -> (37, 12.5)
  line L14 (37, 12.5) -> (37, 14.5)
  line L15 (37, 14.5) -> (41, 14.5)
  line L16 (41, 14.5) -> (41, 15.5)
  line L17 (41, 15.5) -> (35, 15.5)
  line L18 (0.5, 9.5) -> (22.5, 9.5)
  line L19 (22.5, 9.5) -> (22.5, 6.5)
  line L20 (22.5, 6.5) -> (0.5, 6.5)
  line L21 (0.5, 6.5) -> (0.5, 9.5)
  dimension "d209" = 22
  dimension "d210" = 3
  constraint horizontal L18
  constraint vertical L19
  constraint horizontal L20
  constraint vertical L21
  measures "d209" distance of L18.start L18.end
  measures "d210" distance of L18.start L20.end
extrude "拉伸58" cut sketch "草图21" along normal mid plane 74 contours L18 L19 L20 L21 bodies 4
fillet "圆角5" radius 3.5 4 edges at (73, 21, 9.25) (73, -43, 9.25) (100.5, 21, 9.25) (100.5, -43, 9.25) on bodies 4
fillet "圆角6" radius 3.5 4 edges at (100.5, -43, 20) (100.5, 21, 20) (73, 21, 20) (73, -43, 20) on bodies 7
extrude "拉伸59" cut 2 faces at (95.8082, -38.6361, 20.6) (77.2252, 15.9856, 20.6) along direction (0, 0, 1) blind 0.1 on bodies 7 bodies 7
extrude "拉伸60" add 2 faces at (74.3333, -15.1667, 6.5) (99.1667, -15.1667, 6.5) along direction (0, 0, 1) blind 3 on bodies 4 bodies 4
sketch "草图22" plane through (98.5, 0, 0) normal (-1, 0, 0) x (0, -1, 0)
  line L0 (35, 15.5) -> (35, 18.5)
  line L1 (35, 18.5) -> (-19, 18.5)
  line L2 (-19, 18.5) -> (-19, 2)
  line L3 (-19, 2) -> (-12.5, 2)
  line L4 (-12.5, 2) -> (-12.5, 11)
  line L5 (-12.5, 11) -> (-8.2706, 11)
  line L6 (-8.2706, 11) -> (-8.2706, 2)
  line L7 (-8.2706, 2) -> (41, 2)
  line L8 (41, 2) -> (41, 9)
  line L9 (41, 9) -> (37, 9)
  line L10 (37, 9) -> (37, 11)
  line L11 (37, 11) -> (41, 11)
  line L12 (41, 11) -> (41, 12.5)
  line L13 (41, 12.5) -> (37, 12.5)
  line L14 (37, 12.5) -> (37, 14.5)
  line L15 (37, 14.5) -> (41, 14.5)
  line L16 (41, 14.5) -> (41, 15.5)
  line L17 (41, 15.5) -> (35, 15.5)
  line L18 (-1.0855, 10) -> (10.9145, 10)
  line L19 (10.9145, 10) -> (10.9145, 4)
  line L20 (10.9145, 4) -> (-1.0855, 4)
  line L21 (-1.0855, 4) -> (-1.0855, 10)
  line L22 (-2.5855, 7) -> (12.4145, 7) construction
  circle A0 centre (-2.5855, 7) radius 1.118
  circle A1 centre (12.4145, 7) radius 1.2018
  dimension "d221" = 12
  dimension "d222" = 6
  dimension "d223" = 15
  dimension "d224" = 1.5
  constraint horizontal L18
  constraint vertical L19
  constraint horizontal L20
  constraint vertical L21
  constraint perpendicular L19 L22
  constraint coincident L22.start A0.centre
  constraint coincident L22.end A1.centre
  measures "d221" distance of L18.start L18.end
  measures "d222" distance of L18.start L20.end
  measures "d223" distance of L22.start L22.end
  measures "d224" distance of L19 L22.end
extrude "拉伸61" cut sketch "草图22" against normal blind 8 contours L18 L19 L20 L21 | A0 | A1 bodies 4
thread "螺纹3" "ISO Metric profile 2.2 M2.2x0.45 M2.2x0.45 6H" major diameter 2.28 minor diameter 1.7754 pitch 0.45 angle 60 resizes the face on face at (99.1667, 1.473, 6.8887) on face at (99.1667, -13.6104, 6.8803) on bodies 4
sketch "草图23" plane through (0, 0, 21.5) normal (0, 0, 1) x (-1, 0, 0)
  arc A0 (-73, 39.5) -> (-76.5, 43) centre (-76.5, 39.5) ccw
  line L0 (-76.5, 43) -> (-97, 43)
  arc A1 (-97, 43) -> (-100.5, 39.5) centre (-97, 39.5) ccw
  line L1 (-100.5, 39.5) -> (-100.5, -17.5)
  arc A2 (-100.5, -17.5) -> (-97, -21) centre (-97, -17.5) ccw
  line L2 (-97, -21) -> (-76.5, -21)
  arc A3 (-76.5, -21) -> (-73, -17.5) centre (-76.5, -17.5) ccw
  line L3 (-73, -17.5) -> (-73, 39.5)
  line L4 (-81.2, -0.4) -> (-81.2, -6.4)
  line L5 (-81.2, -6.4) -> (-92.8, -6.4)
  line L6 (-92.8, -6.4) -> (-92.8, -0.4)
  line L7 (-92.8, -0.4) -> (-81.2, -0.4)
  line L8 (-73.0321, 3.5866) -> (-100.5391, 3.5866)
  line L9 (-100.5391, 3.5866) -> (-100.5391, 24.5866)
  line L10 (-100.5391, 24.5866) -> (-73.0321, 24.5866)
  line L11 (-73.0321, 24.5866) -> (-73.0321, 3.5866)
  line L12 (-73, 2) -> (-100.5, 2)
  line L13 (-73, 27) -> (-100.5, 27)
  dimension "d229" = 21
  constraint horizontal L8
  constraint vertical L9
  constraint horizontal L10
  constraint vertical L11
  constraint coincident L3 L12.start
  constraint coincident L1 L12.end
  constraint perpendicular L1 L12
  constraint coincident L3 L13.start
  constraint coincident L1 L13.end
  constraint perpendicular L1 L13
  measures "d229" distance of L8.start L10.end
extrude "拉伸62" add sketch "草图23" along normal blind 1.5 contours L1 L3 L8 L10 L11 L12 L13 | L1 L8 L10 L11 bodies 7
extrude "拉伸63" cut sketch "草图23" along normal blind 0.6 and the other way blind 2.2 contours L1 L8 L10 L11 bodies 7
extrude "拉伸64" cut 1 faces at (73.0321, -17.5866, 20.2333) along direction (-1, 0, 0) blind 3 on bodies 7 bodies 7
hidden bodies 1 2 3 5
named bodies: "地板"
